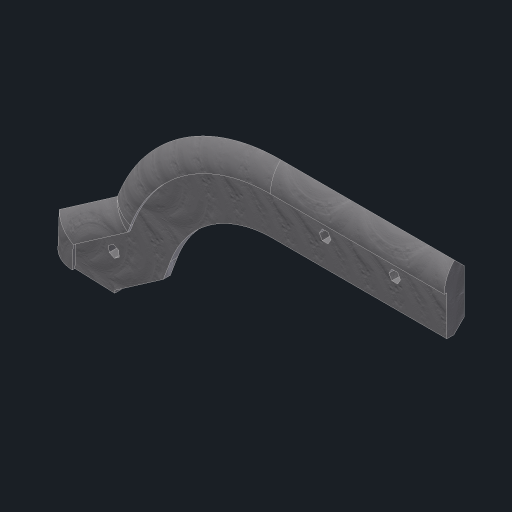
# Autodesk Inventor part: ESQUINA_REDONDEADA_R20
Saved by Autodesk Inventor 2024.3 (Build 283343000, 343)
## iProperties
Created: 2024-05-19
Part Number: ESQUINA_REDONDEADA_R20
Material: Steel, Mild, Welded
Document SubType Name: Modeling
Designer: Niler
Density: 7.85 g/cm^3
Appearance: Weld - Steel Mild
Author: Niler
Autodesk Inventor part; units mm, degrees
ref_plane "YZ Plane" through (0, 0, 0) normal (1, 0, 0) x (0, 1, 0)
ref_plane "XZ Plane" through (0, 0, 0) normal (0, 1, 0) x (-1, 0, 0)
sketch "Sketch1" plane through (0, 0, 0) normal (1, 0, 0) x (0, 1, 0)
  circle A0 centre (0, 0) radius 20
  line L0 (8.5, 8.5) -> (-16.9, 8.5)
  line L1 (8.5, 8.5) -> (8.5, -16.9)
  line L2 (0, 0) -> (0, 20)
  line L3 (0, 20) -> (-60.9241, 20)
  line L4 (-60.9241, 20) -> (-60.9241, 18.5)
  line L5 (-60.9241, 18.5) -> (0, 18.5)
  line L6 (0, 18.5) -> (0, 20)
  line L7 (0, 0) -> (14.1421, 14.1421)
  line L8 (0, 0) -> (20, 0)
  line L9 (-16.9, 8.5) -> (-16.9, 18.5)
  line L10 (-16.9, 8.5) -> (-22.9, 14.5)
  line L11 (-22.9, 14.5) -> (-22.9, 18.5)
  line L12 (12.3744, 12.3744) -> (12.1502, 13.2109)
  line L13 (11.3137, 13.435) -> (9.2071, 11.3284)
  line L14 (9.4313, 10.4919) -> (10.2678, 10.2678)
  line L15 (8.5, 8.5) -> (8.5, -16.9)
  line L16 (20, 0) -> (20, -60.9241)
  line L17 (20, -60.9241) -> (18.5, -60.9241)
  line L18 (18.5, -60.9241) -> (18.5, 0)
  line L19 (8.5, -16.9) -> (18.5, -16.9)
  line L20 (8.5, -16.9) -> (14.5, -22.9)
  line L21 (14.5, -22.9) -> (18.5, -22.9)
  arc A1 (9.2071, 11.3284) -> (9.4313, 10.4919) centre (9.5607, 10.9749) ccw
  arc A2 (12.1502, 13.2109) -> (11.3137, 13.435) centre (11.6673, 13.0815) ccw
  line L22 (10.4311, 10.4311) -> (9.483, 10.6851)
  arc A3 (9.3485, 11.187) -> (9.483, 10.6851) centre (9.5607, 10.9749) ccw
  line L23 (9.3485, 11.187) -> (11.4551, 13.2936)
  arc A4 (11.957, 13.1591) -> (11.4551, 13.2936) centre (11.6673, 13.0815) ccw
  line L24 (11.957, 13.1591) -> (12.2111, 12.2111)
  point P0 (0, 8.5)
  point P1 (-17.7041, 9.3041)
  point P2 (-16.9, 10.6953)
  dimension "d0" = 40
  dimension "d1" = 25.4
  dimension "d2" = 1.5
  dimension "d4" = 45
  dimension "d6" = 45
  dimension "d7" = 4
  dimension "d8" = 10
  dimension "d10" = 2.5
  dimension "d11" = 2.5
  dimension "d12" = 60
  dimension "d13" = 1.5
  dimension "d15" = 0.5
  dimension "d16" = 0.2
  constraints: 50 end point, 11 point on circle, 10 point on line, 6 symmetric about line, 5 centre point, 4 perpendicular, 4 tangent, 3 parallel, 2 equal length, 2 horizontal, 2 vertical, 1 coincident, 1 equal radius, 1 vertical alignment, 4 other
  measures "d0" diameter of A0
  measures "d1" distance of L0.start L1.end
  measures "d2" distance of L4.end L3.end
  measures "d4" angle of L2 L7
  measures "d6" angle of L9 L10
  measures "d7" distance of L10.end L11.end
  measures "d8" distance between parallel lines of L0 L5
  measures "d10" distance of L7.end L12.start
  measures "d11" distance of L0.start L14.end
  measures "d12" angle of L7 L12
  measures "d13" distance between parallel lines of L7 L13
  measures "d15" radius of A1
  measures "d16" distance between parallel lines of L13 L23
extrude "Extrusion1" add sketch "Sketch1" along normal blind 100 contours L7 L12 A2 L13 A1 L14 L0 L2 A0 | L7 L24 A4 L23 A3 L22 L14 A1 L13 A2 L12 | L5 L2 L0 L9 A0 | A0 L9 L5 | L7 L22 A3 L23 A4 L24 | L9 L10 A0 | A0 L10 L11 L5 L9
sketch "Sketch2" plane through (0, -22.9, 18.5) normal (0, 0, 1) x (1, 0, 0)
  line L0 (0, 22.9) -> (0, 0) projected
  line L1 (0, 0) -> (100, 0) projected
  line L2 (100, 22.9) -> (100, 0) projected
  line L3 (0, 22.9) -> (100, 22.9) projected
  line L4 (28.3257, 13.1) -> (26.6514, 16)
  line L5 (26.6514, 16) -> (28.3257, 18.9)
  line L6 (28.3257, 18.9) -> (31.6743, 18.9)
  line L7 (31.6743, 18.9) -> (33.3486, 16)
  line L8 (33.3486, 16) -> (31.6743, 13.1)
  line L9 (31.6743, 13.1) -> (28.3257, 13.1)
  line L10 (0, 6) -> (100, 6) projected
  circle A0 centre (30, 16) radius 1.65
  dimension "d20" = 10
  dimension "d21" = 5.8
  dimension "d22" = 30
  dimension "d25" = 3.3
  constraints: 12 end point, 1 centre point, 1 coincident, 1 horizontal alignment, 13 other
  measures "d20" distance from line of L10 point (30, 16)
  measures "d21" distance between parallel lines of L9 L6
  measures "d22" distance from line of point (30, 16) L0
  measures "d25" diameter of A0
extrude "Extrusion2" cut sketch "Sketch2" against normal blind 6 contours L4 L5 L6 L7 L8 L9 | A0
extrude "Extrusion3" cut sketch "Sketch2" against normal through all contours A0
sketch "Sketch3" plane through (0, -22.9, 18.5) normal (0, 0, 1) x (1, 0, 0)
  line L0 (0, 37.0421) -> (100, 37.0421) projected
  line L1 (0, 0) -> (100, 0) projected
  line L2 (0, 22.9) -> (0, 0) projected
  line L3 (0, 22.9) -> (0, 37.0421) projected
  line L4 (2.4384, 37.0421) -> (17.8575, 0)
  line L5 (0, 0) -> (100, 0) projected
  line L6 (2.4384, 37.0421) -> (0, 42.9) projected
  point P0 (0, 26.9698)
  dimension "d28" = 112.6
  constraints: 2 end point, 1 point on line
  measures "d28" angle of L4 L0
sketch "Sketch4" plane through (100, 14.1421, 14.1421) normal (0, 0.7071068, -0.7071068) x (-1, 0, 0)
  line L0 (100, 0) -> (0, 0) projected
  line L1 (0, -7.9792) -> (0, 0) projected
  line L2 (100, -7.9792) -> (0, -7.9792) projected
  circle A0 centre (80, -4) radius 1.5
  line L3 (100, -7.9792) -> (100, 0) projected
  line L4 (50, -7.9792) -> (50, 0)
  ellipse E0 centre (70, -18.8686) end of major axis (68.35, -18.8686) minor radius 1.1667 projected
  point P0 (100, -20)
  dimension "d34" = 3
  dimension "d35" = 4
  dimension "d46" = 20
  constraints: 2 end point, 2 midpoint, 1 centre point, 1 other
  measures "d34" diameter of A0
  measures "d35" distance from line of L0 A0.centre
  measures "d46" distance from line of L3 A0.centre
extrude "Extrusion5" cut sketch "Sketch4" against normal blind 3 contours A0
ref_plane "Work Plane1" through (50, 0, 0) normal (-1, 0, 0) x (0, 0, 1)
mirror "Mirror1" about plane through (50, 0, 0) normal (-1, 0, 0) of "Extrusion5", "Extrusion2", "Extrusion3"
ref_plane "Work Plane2" through (0, 14.1421, 14.1421) normal (0, 0, 1) x (1, 0, 0)
sketch "Sketch9" plane through (0, 14.1421, 14.1421) normal (0, 0, 1) x (1, 0, 0)
  line L0 (0, 0) -> (100, 0) projected
  line L1 (0, 0) -> (-127.2781, -88.4606) construction
  line L2 (0, -14.1421) -> (0, 0) projected
  arc A0 (0, 0) -> (-93.7282, -65.1428) centre (0, -100) ccw
  line L3 (-127.2781, -88.4606) -> (-93.7282, -65.1428)
  line L4 (-127.2781, -88.4606) -> (-128.0459, -108.4459)
  dimension "d61" = 155
  dimension "d62" = 145.2
  dimension "d63" = 100
  dimension "d66" = 127
  dimension "d67" = 20
  constraints: 6 end point, 2 point on circle, 1 centre point, 1 collinear, 1 point on line, 1 tangent
  measures "d61" distance of L0.start L1.end
  measures "d62" angle of L0 L1
  measures "d63" radius of A0
  measures "d66" angle of L4 L1
  measures "d67" distance of L1.end L4.end
sketch "Sketch10" plane through (0, 0, 0) normal (-1, 0, 0) x (0, 0, 1)
  line L0 (14.5, -22.9) -> (8.5, -16.9) projected
  line L1 (18.5, -22.9) -> (14.5, -22.9) projected
  line L2 (18.5, 0) -> (18.5, -22.9) projected
  line L3 (20, 0) -> (18.5, 0) projected
  arc A0 (20, 0) -> (14.1421, 14.1421) centre (0, 0) ccw projected
  line L4 (8.5, 8.5) -> (14.1421, 14.1421) projected
  line L5 (8.5, -16.9) -> (8.5, 8.5) projected
sweep "Sweep2" add profiles "Sketch10" path "Sketch9" path curves A0 L3 L4
sketch "Sketch11" plane through (100, -22.9, 18.5) normal (0, 0, 1) x (1, 0, 0)
  line L0 (-33.3486, 16) -> (-31.6743, 18.9) projected
  line L1 (-31.6743, 18.9) -> (-28.3257, 18.9) projected
  line L2 (-28.3257, 18.9) -> (-26.6514, 16) projected
  line L3 (-26.6514, 16) -> (-28.3257, 13.1) projected
  line L4 (-28.3257, 13.1) -> (-31.6743, 13.1) projected
  line L5 (-31.6743, 13.1) -> (-33.3486, 16) projected
  line L6 (-68.3257, 18.9) -> (-66.6514, 16) projected
  line L7 (-66.6514, 16) -> (-68.3257, 13.1) projected
  line L8 (-68.3257, 13.1) -> (-71.6743, 13.1) projected
  line L9 (-71.6743, 13.1) -> (-73.3486, 16) projected
  line L10 (-73.3486, 16) -> (-71.6743, 18.9) projected
  line L11 (-71.6743, 18.9) -> (-68.3257, 18.9) projected
  line L12 (-100, 0) -> (0, 0) projected
  line L13 (-100, 22.9) -> (0, 22.9) projected
  arc A0 (-100, 22.9) -> (-180.473, -33.0302) centre (-100, -62.9579) ccw projected
  line L14 (-180.473, -33.0302) -> (-182.0179, -37.1841) projected
  line L15 (-182.0179, -37.1841) -> (-213.4171, -59.0072) projected
  line L16 (-213.4171, -59.0072) -> (-213.9142, -71.9466) projected
  line L17 (-190.9723, -71.2953) -> (-191.0311, -72.8257) projected
  line L18 (-163.0556, -51.8928) -> (-190.9723, -71.2953) projected
  line L19 (-159.0093, -41.0125) -> (-163.0556, -51.8928) projected
  arc A1 (-100, 0) -> (-159.0093, -41.0125) centre (-100, -62.9579) ccw projected
  circle A2 centre (-30, 16) radius 1.65 projected
  circle A3 centre (-70, 16) radius 1.65 projected
  line L20 (-100, 31.4) -> (0, 31.4) projected
  line L21 (-100, 6) -> (0, 6) projected
  arc A4 (-100, 6) -> (-164.633, -38.9211) centre (-100, -62.9579) ccw projected
  line L22 (-164.633, -38.9211) -> (-168.0239, -48.039) projected
  line L23 (-168.0239, -48.039) -> (-196.853, -68.0757) projected
  line L24 (-196.853, -68.0757) -> (-197.0266, -72.5954) projected
  line L25 (-221.7481, -54.446) -> (-222.4079, -71.6203) projected
  line L26 (-189.0563, -31.7246) -> (-221.7481, -54.446) projected
  line L27 (-188.4399, -30.0674) -> (-189.0563, -31.7246) projected
  arc A5 (-100, 31.4) -> (-188.4399, -30.0674) centre (-100, -62.9579) ccw projected
  line L28 (-207.0193, -72.2115) -> (-206.6542, -62.7097)
  line L29 (-206.6542, -62.7097) -> (-176.3043, -41.616)
  line L30 (-176.3043, -41.616) -> (-174.0058, -35.4354)
  arc A6 (-100, 16) -> (-174.0058, -35.4354) centre (-100, -62.9579) ccw
  line L31 (-100, 16) -> (0, 16)
  circle A7 centre (-191.4793, -52.1629) radius 1.65
  line L32 (-194.229, -54.074) -> (-194.5092, -50.7371)
  line L33 (-194.5092, -50.7371) -> (-191.7595, -48.826)
  line L34 (-191.7595, -48.826) -> (-188.7296, -50.2517)
  line L35 (-188.7296, -50.2517) -> (-188.4494, -53.5886)
  line L36 (-188.4494, -53.5886) -> (-191.1991, -55.4997)
  line L37 (-191.1991, -55.4997) -> (-194.229, -54.074)
  point P0 (-189.8242, -54.5442)
  dimension "d68" = 10
  dimension "d69" = 3.3
  dimension "d70" = 5.8
  constraints: 20 end point, 8 centre point, 2 midpoint, 2 point on circle, 1 coincident, 1 point on line, 17 other
  measures "d68" distance between parallel lines of L22 L30
  measures "d69" diameter of A7
  measures "d70" distance from line of L33 point (-189.824, -54.544)
extrude "Extrusion7" cut sketch "Sketch11" against normal through all contours A7 L29 | L29 A7
extrude "Extrusion8" cut sketch "Sketch11" against normal blind 6 contours L32 L33 L34 L29 A7 | L29 A7 L35 L36 L37 | A7 L29 | L29 A7
body "Solid1"
